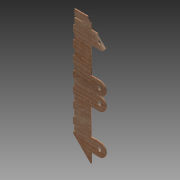
# Autodesk Inventor part: zijiplaaten
Saved by Autodesk Inventor 2015 (Build 190159000, 159)
## iProperties
Created: 2015-12-19
Part Number: zijiplaaten
Material: Generic
Document SubType Name: Modeling
Designer: david
Density: 1 g/cm^3
Appearance: Birch - Natural Polished
Mass: 76.8496 g
Surface Area: 553.968 cm^2
Volume: 76.8496 cm^3
Author: david
Autodesk Inventor part; units mm, degrees
ref_plane "YZ Plane" through (0, 0, 0) normal (1, 0, 0) x (0, 1, 0)
ref_plane "XZ Plane" through (0, 0, 0) normal (0, 1, 0) x (-1, 0, 0)
ref_plane "XY Plane" through (0, 0, 0) normal (0, 0, 1) x (1, 0, 0)
sketch "Sketch1" plane through (0, 0, 0) normal (0, 1, 0) x (-1, 0, 0)
  line L0 (-25, 190) -> (25, 190)
  line L1 (25, 190) -> (25, -190)
  line L2 (25, -190) -> (-25, -190)
  line L3 (-25, -190) -> (-25, 190)
  line L4 (-25, 190) -> (25, -190) construction
  line L5 (25, 190) -> (-25, -190) construction
  point P0 (0, 0)
  dimension "d0" = 50
  dimension "d1" = 380
  constraints: 12 end point, 2 midpoint, 2 parallel, 1 horizontal, 1 perpendicular
  measures "d0" distance of L1.end L2.end
  measures "d1" distance of L0.end L1.end
extrude "Extrusion1" add sketch "Sketch1" along normal blind 3
sketch "Sketch2" plane through (0, 3, 0) normal (0, 1, 0) x (1, 0, 0)
  line L0 (25, -160) -> (50, -160)
  line L1 (50, -160) -> (50, -120)
  line L2 (50, -120) -> (25, -120)
  line L3 (25, -120) -> (25, -160)
  line L4 (50, -40) -> (20, -40)
  line L5 (20, -40) -> (20, 40)
  line L6 (20, 40) -> (50, 40)
  line L7 (50, 40) -> (50, -40)
  line L8 (50, -40) -> (20, 40) construction
  line L9 (20, -40) -> (50, 40) construction
  line L10 (30, 160) -> (50, 160)
  line L11 (50, 160) -> (50, 120)
  line L12 (50, 120) -> (30, 120)
  line L13 (30, 120) -> (30, 160)
  circle A0 centre (50, -140) radius 20
  circle A1 centre (50, -20) radius 20
  circle A2 centre (50, 20) radius 20
  circle A3 centre (50, 140) radius 20
  line L14 (25, 190) -> (25, -190) projected
  line L15 (25, -190) -> (25, 190) projected
  line L16 (30, 160) -> (25, 160)
  line L17 (25, 160) -> (25, 120)
  line L18 (25, 120) -> (30, 120)
  line L19 (30, 120) -> (30, 160)
  line L20 (25, -120) -> (25, -120)
  line L21 (25, -120) -> (25, -150)
  line L22 (25, -150) -> (25, -150)
  line L23 (25, -150) -> (25, -120)
  line L24 (50, 0) -> (35, 0)
  line L25 (35, 0) -> (35, 5)
  line L26 (35, 5) -> (50, 5)
  line L27 (50, 5) -> (50, 0)
  line L28 (25, 190) -> (-25, 190) projected
  line L29 (-25, -190) -> (25, -190) projected
  point P0 (0, 0)
  point P1 (35, 0)
  dimension "d10" = 40
  dimension "d4" = 25
  dimension "d5" = 40
  dimension "d7" = 80
  dimension "d8" = 20
  dimension "d9" = 40
  dimension "d11" = 40
  dimension "d12" = 20
  dimension "d13" = 20
  dimension "d16" = 80
  dimension "d17" = 80
  dimension "d18" = 5
  dimension "d19" = 25
  dimension "d20" = 25
  dimension "d40" = 15
  dimension "d41" = 30
  dimension "d43" = 70
  dimension "d44" = 40
  dimension "d49" = 70
  constraints: 52 end point, 12 equal length, 6 horizontal, 6 perpendicular, 5 midpoint, 4 point on line, 3 vertical alignment, 1 centre point, 6 other
  measures "d4" distance of L2.end L1.end
  measures "d5" distance of L1.end L0.end
  measures "d7" distance of L4.end L5.end
  measures "d8" distance of L11.end L12.end
  measures "d9" distance of L10.end L11.end
  measures "d11" diameter of A2
  measures "d12" distance from line of L4 point (50, -20)
  measures "d13" distance from line of L6 A2.centre
  measures "d16" distance between parallel lines of L6 L12
  measures "d17" distance between parallel lines of L4 L2
  measures "d18" distance between parallel lines of L14 L13
  measures "d19" distance between parallel lines of L14 L7
  measures "d20" distance between parallel lines of L14 L1
  measures "d40" distance of L25.end L26.end
  measures "d41" distance between parallel lines of L20 L22
  measures "d43" distance between parallel lines of L28 L12
  measures "d44" distance between parallel lines of L16 L18
  measures "d49" distance between parallel lines of L29 L20
extrude "Extrusion2" add sketch "Sketch2" against normal blind 3
sketch "Sketch3" plane through (0, 3, 0) normal (0, 1, 0) x (1, 0, 0)
  line L0 (-25, 190) -> (-25, -190) projected
  line L1 (-25, -167.5) -> (0, -167.5)
  line L2 (0, -167.5) -> (0, -171.5)
  line L3 (0, -171.5) -> (-25, -171.5)
  line L4 (-25, -171.5) -> (-25, -167.5)
  line L5 (25, -190) -> (-25, -190) projected
  line L6 (-25, 171.5) -> (0, 171.5)
  line L7 (0, 171.5) -> (0, 167.5)
  line L8 (0, 167.5) -> (-25, 167.5)
  line L9 (-25, 167.5) -> (-25, 171.5)
  line L10 (-25, 190) -> (25, 190) projected
  point P0 (0, 0)
  dimension "d21" = 25
  dimension "d22" = 4
  dimension "d23" = 18.5
  dimension "d26" = 4
  dimension "d27" = 18.5
  dimension "d50" = 25
  constraints: 16 end point, 4 parallel, 2 horizontal, 2 perpendicular, 2 point on line
  measures "d21" distance of L2.end L3.end
  measures "d22" distance of L1.end L2.end
  measures "d23" distance between parallel lines of L5 L3
  measures "d26" distance of L6.end L7.end
  measures "d27" distance between parallel lines of L10 L6
  measures "d50" distance of L7.end L8.end
extrude "Extrusion3" cut sketch "Sketch3" against normal blind 3
sketch "Sketch4" plane through (0, 0, 0) normal (0, -1, 0) x (1, 0, 0)
  circle A0 centre (50, -20) radius 5.15
  arc A1 (50, -40) -> (50, 0) centre (50, -20) ccw projected
  circle A2 centre (50, 20) radius 5.15
  line L0 (25, 40) -> (50, 40) projected
  circle A3 centre (50, -140) radius 5.15
  line L1 (50, -120) -> (25, -120) projected
  arc A4 (50, -160) -> (50, -120) centre (50, -140) ccw projected
  circle A5 centre (50, 140) radius 5.15
  line L2 (50, 160) -> (25, 160) projected
  arc A6 (50, 120) -> (50, 160) centre (50, 140) ccw projected
  point P0 (0, 0)
  point P1 (25, 160)
  point P2 (25, 290)
  dimension "d28" = 10.3
  dimension "d30" = 0
  dimension "d31" = 10.3
  dimension "d33" = 10.3
  dimension "d36" = 10.3
  dimension "d42" = 40
  dimension "d51" = 0
  dimension "d52" = 0
  constraints: 4 centre point, 1 other
  measures "d28" diameter of A0
  measures "d30" distance of A1.centre A0.centre
  measures "d31" diameter of A2
  measures "d33" diameter of A3
  measures "d36" diameter of A5
  measures "d42" distance of A2.centre A0.centre
  measures "d51" distance of A6.centre A5.centre
  measures "d52" distance of A4.centre A3.centre
extrude "Extrusion4" cut sketch "Sketch4" against normal blind 10
sketch "Sketch6" plane through (0, 0, 0) normal (0, -1, 0) x (1, 0, 0)
  line L0 (-25, 167.5) -> (-25, -167.5) projected
  line L1 (-25, 167.5) -> (0, 167.5) projected
  line L2 (-21, 147.5) -> (-28, 147.5)
  line L3 (-29, 146.5) -> (-29, 128.5)
  line L4 (-28, 127.5) -> (-21, 127.5)
  line L5 (-21, 127.5) -> (-21, 147.5)
  line L6 (-25, -167.5) -> (-25, 167.5) projected
  line L7 (-21, 147.5) -> (-29, 127.5) construction
  line L8 (-29, 147.5) -> (-21, 127.5) construction
  arc A0 (-28, 147.5) -> (-29, 146.5) centre (-28, 146.5) ccw
  arc A1 (-29, 128.5) -> (-28, 127.5) centre (-28, 128.5) ccw
  point P0 (0, 0)
  point P1 (-25, 137.5)
  dimension "d54" = 8
  dimension "d55" = 20
  dimension "d56" = 1
  dimension "d57" = 20
  constraints: 12 end point, 5 point on line, 4 point on circle, 4 tangent, 2 centre point, 2 midpoint, 2 parallel, 1 equal radius, 1 horizontal, 1 perpendicular
  measures "d54" distance of L4.end L7.end
  measures "d55" distance of L7.end L8.start
  measures "d56" radius of A0
  measures "d57" distance between parallel lines of L1 L2
extrude "Extrusion5" add sketch "Sketch6" against normal blind 3
pattern_linear "Rectangular Pattern1" count 8 spacing 40 along (0, 0, -1) of "Extrusion5"
body "Solid1"
